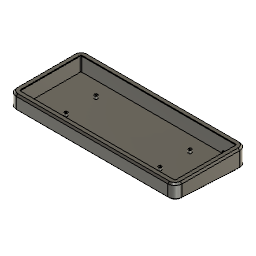
CNC QAZ MFR2 (Autodesk Fusion 360 design; units mm, degrees)
Autodesk Fusion 360 part; units mm, degrees
sketch "PCB Plane" plane through (0, 0, 0) normal (0, 0, 1) x (1, 0, 0)
  line L0 (0, 0) -> (195.263, 0) construction
  line L1 (195.263, 0) -> (195.263, 76.2) construction
  line L2 (195.263, 76.2) -> (0, 76.2) construction
  line L3 (0, 76.2) -> (0, 0) construction
  line L4 (-0.5, -0.5) -> (195.763, -0.5)
  line L5 (195.763, -0.5) -> (195.763, 76.7)
  line L6 (195.763, 76.7) -> (-0.5, 76.7)
  line L7 (-0.5, 76.7) -> (-0.5, -0.5)
  line L8 (-7.5, 83.7) -> (-7.5, -7.5)
  line L9 (-7.5, -7.5) -> (202.763, -7.5)
  line L10 (202.763, -7.5) -> (202.763, 83.7)
  line L11 (202.763, 83.7) -> (-7.5, 83.7)
  dimension "d1" = 195.263
  dimension "d2" = 76.2
  dimension "d3" = 0.5
  dimension "d4" = 7.5
  constraint horizontal L0
  constraint vertical L1
  constraint horizontal L2
  constraint vertical L3
  constraint coincident L0.start L3.end
  measures "d1" distance of L0.start L0.end
  measures "d2" distance of L0.start L2.end
ref_plane "WorkPlane1" through (97.6315, 38.1, -3.46) normal (0, 0, 1) x (1, 0, 0)
ref_plane "WorkPlane2" through (97.6315, 38.1, 14.6) normal (0, 0, 1) x (1, 0, 0)
extrude "Extrude1" add sketch "PCB Plane" along normal up to surface (14.6 mm away) and the other way up to surface (3.46 mm away)
sketch "Angle Sketch" plane through (202.763, 0, 0) normal (1, 0, 0) x (0, 1, 0)
  line L0 (83.7, 14.6) -> (-7.5, 14.6)
  line L1 (-7.5, 14.6) -> (-7.5, -3.46)
  line L2 (-7.5, -3.46) -> (83.7, -3.46)
  line L3 (83.7, -3.46) -> (83.7, 14.6)
  line L4 (-7.5, 14.6) -> (-7.5, -3.6755)
  line L5 (-7.5, -3.6755) -> (92.363, -8.9091)
  line L6 (-7.5, -3.6755) -> (92.5, -3.6755) construction
  dimension "d11" = 18.2755
  dimension "d12" = 100
  dimension "d13" = 3
  constraint coincident L0.end L1.start
  constraint perpendicular L0 L4
  constraint horizontal L6
  measures "d11" distance of L0.end L4.end
  measures "d12" distance of L4.end L5.end
  measures "d13" angle of L5 L6
ref_plane "WorkPlane3" through (202.763, 42.4315, -6.2923) normal (0, -0.052336, -0.99863) x (0, 0.99863, -0.052336)
sketch "Interior Base Plane" plane through (0, 0, -3.46) normal (0, 0, -1) x (1, 0, 0)
  line L0 (195.763, -76.7) -> (-0.5, -76.7)
  line L1 (-0.5, -76.7) -> (-0.5, 0.5)
  line L2 (-0.5, 0.5) -> (195.763, 0.5)
  line L3 (195.763, 0.5) -> (195.763, -76.7)
  line L4 (-7.5, 7.5) -> (-7.5, -83.7)
  line L5 (-7.5, -83.7) -> (202.763, -83.7)
  line L6 (202.763, -83.7) -> (202.763, 7.5)
  line L7 (202.763, 7.5) -> (-7.5, 7.5)
  line L8 (-7.5, 7.5) -> (202.763, 7.5)
  line L9 (202.763, 7.5) -> (202.763, -83.7)
  line L10 (202.763, -83.7) -> (-7.5, -83.7)
  line L11 (-7.5, -83.7) -> (-7.5, 7.5)
  constraint horizontal L8
  constraint vertical L9
  constraint horizontal L10
  constraint vertical L11
  constraint coincident L5.end L6.start
  constraint coincident L4.start L7.end
extrude "Extrude2" add sketch "Interior Base Plane" along normal up to surface contours L0 L1 L2 L3 | L4 L5 L6 L7 L8 L9 L10 L11 end surface through (202.763, 42.4315, -6.2923) normal (0, -0.052336, -0.99863) offset 0
fillet "Fillet1" radius 9 1 edges at (202.763, -7.5, 5.4623)
fillet "Fillet2" radius 9 1 edges at (202.763, 83.7, 3.0725)
fillet "Fillet3" radius 9 1 edges at (-7.5, 83.7, 3.0725)
fillet "Fillet4" radius 9 1 edges at (-7.5, -7.5, 5.4623)
fillet "Fillet5" radius 1 1 edges at (195.763, 76.7, 5.57)
fillet "Fillet6" radius 1 1 edges at (-0.5, 76.7, 5.57)
fillet "Fillet7" radius 1 1 edges at (195.763, -0.5, 5.57)
fillet "Fillet8" radius 1 1 edges at (-0.5, -0.5, 5.57)
chamfer "Chamfer1" distance 2 angle 45 8 edges at (-7.5, 38.1, 14.6) (-4.864, 81.064, 14.6) (97.6315, 83.7, 14.6) (200.127, 81.064, 14.6) (202.763, 38.1, 14.6) (200.127, -4.864, 14.6) (97.6315, -7.5, 14.6) (-4.864, -4.864, 14.6)
chamfer "Chamfer2" distance 2 angle 45 8 edges at (-7.5, 38.1, -6.0653) (-4.864, -4.864, -3.8136) (97.6315, -7.5, -3.6755) (200.127, -4.864, -3.8136) (202.763, 38.1, -6.0653) (200.127, 81.064, -8.3169) (97.6315, 83.7, -8.4551) (-4.864, 81.064, -8.3169)
chamfer "Chamfer3" distance 0.5 angle 45 4 edges at (97.6315, 76.7, 14.6) (-0.5, 38.1, 14.6) (97.6315, -0.5, 14.6) (195.763, 38.1, 14.6)
extrude "Extrude3" add 1 faces at (129.6753, 23.5658, -5.3036) along direction (0, 0.052336, 0.99863) blind 1
ref_plane "WorkPlane4" through (97.6315, 38.1, 0) normal (0, 0, 1) x (1, 0, 0)
sketch "USB C Hole Internal" plane through (0, 76.7, 0) normal (0, -1, 0) x (1, 0, 0)
  line L0 (194.763, 14.1) -> (0.5, 14.1)
  line L1 (0.5, -3.46) -> (194.763, -3.46)
  line L2 (180.1818, -3.46) -> (186.5317, -3.46)
  line L3 (188.0818, -1.91) -> (188.0818, -1.35)
  line L4 (186.5318, 0.2) -> (180.1818, 0.2)
  line L5 (178.6318, -1.35) -> (178.6318, -1.91)
  arc A0 (180.1818, 0.2) -> (178.6318, -1.35) centre (180.1818, -1.35) ccw
  arc A1 (188.0818, -1.35) -> (186.5318, 0.2) centre (186.5318, -1.35) ccw
  arc A2 (186.5318, -3.46) -> (188.0818, -1.91) centre (186.5318, -1.91) ccw
  arc A3 (178.6318, -1.91) -> (180.1818, -3.46) centre (180.1818, -1.91) ccw
  line L6 (0.5, 14.1) -> (0.5, -3.46)
  line L7 (194.763, -3.46) -> (194.763, 14.1)
  line L8 (194.763, -0.2545) -> (195.263, -0.2545)
  line L9 (183.3568, 0.2) -> (183.3568, -3.46) construction
  dimension "d36" = 1.55
  dimension "d82" = 0.5
  dimension "d83" = 4.725
  dimension "d84" = 11.9062
  dimension "d89" = 3.66
  dimension "d90" = 3.66
  constraint horizontal L2
  constraint vertical L3
  constraint horizontal L4
  constraint vertical L5
  constraint tangent L5 A0
  constraint tangent L4 A0
  constraint tangent L4 A1
  constraint tangent L3 A1
  constraint equal A0 A1
  constraint tangent L2 A2
  constraint tangent L3 A2
  constraint equal A0 A2
  constraint tangent L2 A3
  constraint tangent L5 A3
  constraint equal A0 A3
  constraint coincident L7 L8.start
  constraint perpendicular L7 L8
  constraint midpoint L4 L9.start
  constraint midpoint L2 L9.end
  measures "d36" radius of A0
  measures "d82" distance of L8.start L8.end
  measures "d83" distance of L5 L9
  measures "d84" distance of L8.end L9
  measures "d89" distance of L2 L4
  measures "d90" distance of L1 L4
extrude "Extrude4" cut sketch "USB C Hole Internal" against normal through all contours L1 L2 L3 L4 L5 A0 A1 A2 A3
sketch "USB C Hole External" plane through (0, 83.7, 0) normal (0, 1, 0) x (-1, 0, 0)
  line L0 (-186.5318, 0.2) -> (-180.1818, 0.2)
  arc A0 (-178.6318, -1.35) -> (-180.1818, 0.2) centre (-180.1817, -1.35) ccw
  line L1 (-178.6318, -1.35) -> (-178.6318, -1.91)
  arc A1 (-180.1818, -3.46) -> (-178.6317, -1.91) centre (-180.1817, -1.91) ccw
  line L2 (-180.1818, -3.46) -> (-186.5317, -3.46)
  arc A2 (-188.0818, -1.91) -> (-186.5318, -3.46) centre (-186.5318, -1.91) ccw
  line L3 (-188.0818, -1.91) -> (-188.0818, -1.35)
  arc A3 (-186.5318, 0.2) -> (-188.0818, -1.35) centre (-186.5318, -1.35) ccw
  line L4 (-193.763, -6.4551) -> (-1.5, -6.4551)
  line L5 (-1.5, -6.4551) -> (-1.5, 12.6)
  line L6 (-1.5, 12.6) -> (-193.763, 12.6)
  line L7 (-193.763, 12.6) -> (-193.763, -6.4551)
  line L8 (-178.6318, -1.63) -> (-188.0817, -1.63) construction
  line L9 (-183.3568, 0.2) -> (-183.3568, -3.46) construction
  line L10 (-183.8568, 2.45) -> (-183.8568, -5.71) construction
  line L11 (-190.8318, -1.63) -> (-176.8818, -1.63) construction
  line L12 (-186.5318, 2.45) -> (-180.1818, 2.45)
  line L13 (-176.3818, -1.35) -> (-176.3818, -1.91)
  line L14 (-180.1818, -5.71) -> (-186.5318, -5.71)
  line L15 (-190.3318, -1.91) -> (-190.3318, -1.35)
  arc A4 (-190.3318, -1.91) -> (-186.5318, -5.71) centre (-186.5318, -1.91) ccw
  arc A5 (-186.5318, 2.45) -> (-190.3318, -1.35) centre (-186.5318, -1.35) ccw
  arc A6 (-176.3818, -1.35) -> (-180.1818, 2.45) centre (-180.1818, -1.35) ccw
  arc A7 (-180.1818, -5.71) -> (-176.3818, -1.91) centre (-180.1818, -1.91) ccw
  dimension "d39" = 8.16
  dimension "d40" = 4.08
  dimension "d42" = 13.95
  dimension "d43" = 3.8
  dimension "d85" = 13.95
  dimension "d86" = 8.16
  dimension "d87" = 6.975
  dimension "d88" = 4.08
  constraint midpoint L1 L8.start
  constraint midpoint L0 L9.start
  constraint midpoint L2 L9.end
  constraint perpendicular L2 L10
  constraint perpendicular L10 L11
  constraint horizontal L12
  constraint vertical L13
  constraint horizontal L14
  constraint vertical L15
  constraint tangent L14 A4
  constraint tangent L15 A4
  constraint tangent L15 A5
  constraint tangent L12 A5
  constraint equal A4 A5
  constraint tangent L12 A6
  constraint tangent L13 A6
  constraint equal A4 A6
  constraint tangent L13 A7
  constraint tangent L14 A7
  constraint equal A4 A7
  measures "d39" distance of L10.start L10.end
  measures "d40" distance of L8 L10.start
  measures "d42" distance of L11.start L11.end
  measures "d43" radius of A4
  measures "d85" distance of L13 L15
  measures "d86" distance of L12 L14
  measures "d87" distance of L9 L15
extrude "Extrude5" cut sketch "USB C Hole External" against normal blind 4.5025 contours L12 L13 L14 L15 A4 A5 A6 A7
chamfer "Chamfer4" distance 0.25 angle 45 8 edges at (189.2188, 83.7, -4.597) (190.3318, 83.7, -1.63) (189.2188, 83.7, 1.337) (183.3568, 83.7, 2.45) (177.4947, 83.7, 1.337) (176.3818, 83.7, -1.63) (177.4947, 83.7, -4.597) (183.3568, 83.7, -5.71)
sketch "Hole Tops" plane through (0, 0, 0) normal (0, 0, 1) x (1, 0, 0)
  line L0 (0, 0) -> (195.2625, 0) construction
  line L1 (195.2625, 0) -> (195.2625, 76.2) construction
  line L2 (195.2625, 76.2) -> (0, 76.2) construction
  line L3 (0, 76.2) -> (0, 0) construction
  line L4 (195.2625, 76.2) -> (195.2625, 57.15) construction
  line L5 (195.2625, 57.15) -> (193.1449, 57.15) construction
  circle A0 centre (157.1625, 57.15) radius 2
  circle A1 centre (38.1, 57.15) radius 2
  circle A2 centre (38.1, 19.05) radius 2
  circle A3 centre (157.1625, 19.05) radius 2
  dimension "d47" = 195.2625
  dimension "d48" = 76.2
  dimension "d51" = 19.05
  dimension "d52" = 38.1
  dimension "d53" = 19.05
  dimension "d54" = 38.1
  dimension "d55" = 38.1
  dimension "d56" = 19.05
  dimension "d57" = 38.1
  dimension "d58" = 19.05
  dimension "d59" = 4
  constraint horizontal L0
  constraint vertical L1
  constraint horizontal L2
  constraint vertical L3
  constraint coincident L0.start L3.end
  constraint perpendicular L2 L4
  constraint perpendicular L1 L5
  constraint equal A0 A1
  constraint equal A0 A3
  constraint equal A1 A2
  measures "d47" distance of L0.start L0.end
  measures "d48" distance of L0.start L2.end
  measures "d51" distance of L2 A0.centre
  measures "d52" distance of L1 A0.centre
  measures "d53" distance of L0 A3.centre
  measures "d54" distance of L1 A3.centre
  measures "d55" distance of L3 A2.centre
  measures "d56" distance of L0 A2.centre
  measures "d57" distance of L3 A1.centre
  measures "d58" distance of L2 A1.centre
  measures "d59" diameter of A1
extrude "Extrude6" add sketch "Hole Tops" against normal up to surface (3.46 mm away)
hole "Hole1" at (157.1625, 19.05, 0) direction (0, 0, -1) diameter 1.6 depth 4 tip angle 180
hole "Hole2" at (157.1625, 57.15, 0) direction (0, 0, -1) diameter 1.6 depth 4 tip angle 180
hole "Hole3" at (38.1, 19.05, 0) direction (0, 0, -1) diameter 1.6 depth 4 tip angle 180
hole "Hole4" at (38.1, 57.15, 0) direction (0, 0, -1) diameter 1.6 depth 4 tip angle 180
sketch "Sketch11" plane through (0, -0.2126, -4.0574) normal (0, -0.052336, -0.99863) x (1, 0, 0)
  line L0 (200.763, -74.9106) -> (200.763, -1.715)
  spline S0 degree 3 poles (200.7625, -1.6334) (200.7627, -1.647) (200.7628, -1.6606) (200.763, -1.6878) (200.763, -1.7014) (200.763, -1.715) knots 1.559167 1.559167 1.559167 1.559167 1.564981 1.564981 1.570796 1.570796 1.570796 1.570796
  spline S1 degree 3 poles (193.763, 5.2974) (194.9008, 5.2974) (196.0377, 5.0141) (197.6563, 4.154) (198.2207, 3.7362) (198.7118, 3.2445) (199.2028, 2.7527) (199.6203, 2.1873) (200.467, 0.5894) (200.7496, -0.52) (200.7625, -1.6334) knots 0 0 0 0 0.48784 0.48784 0.785398 0.785398 0.785398 1.082956 1.082956 1.559167 1.559167 1.559167 1.559167
  line L1 (193.763, 5.2974) -> (1.5, 5.2974)
  spline S2 degree 3 poles (-5.4995, -1.6334) (-5.4866, -0.52) (-5.204, 0.5894) (-4.3573, 2.1873) (-3.9398, 2.7527) (-3.4488, 3.2445) (-2.9577, 3.7362) (-2.3933, 4.154) (-0.7747, 5.0141) (0.3622, 5.2974) (1.5, 5.2974) knots -1.559167 -1.559167 -1.559167 -1.559167 -1.082956 -1.082956 -0.785398 -0.785398 -0.785398 -0.48784 -0.48784 0 0 0 0
  spline S3 degree 3 poles (-5.5, -1.715) (-5.5, -1.7014) (-5.5, -1.6878) (-5.4998, -1.6606) (-5.4997, -1.647) (-5.4995, -1.6334) knots -1.570796 -1.570796 -1.570796 -1.570796 -1.564981 -1.564981 -1.559167 -1.559167 -1.559167 -1.559167
  line L2 (-5.5, -1.715) -> (-5.5, -74.9106)
  line L3 (-5.5, -75.0154) -> (-5.5, -74.9106)
  spline S4 degree 3 poles (1.5, -82.0278) (0.3678, -82.0278) (-0.7633, -81.7474) (-2.384, -80.8913) (-2.9537, -80.4706) (-3.4488, -79.9749) (-3.9439, -79.4791) (-4.3641, -78.9085) (-5.2196, -77.2845) (-5.5, -76.1504) (-5.5, -75.0154) knots 0 0 0 0 0.485398 0.485398 0.785398 0.785398 0.785398 1.085398 1.085398 1.570796 1.570796 1.570796 1.570796
  line L4 (1.5, -82.0278) -> (193.763, -82.0278)
  spline S5 degree 3 poles (200.763, -75.0154) (200.763, -76.1504) (200.4826, -77.2845) (199.6271, -78.9085) (199.2069, -79.4791) (198.7118, -79.9749) (198.2167, -80.4706) (197.647, -80.8913) (196.0263, -81.7474) (194.8952, -82.0278) (193.763, -82.0278) knots -1.570796 -1.570796 -1.570796 -1.570796 -1.085398 -1.085398 -0.785398 -0.785398 -0.785398 -0.485398 -0.485398 0 0 0 0
  line L5 (200.763, -74.9106) -> (200.763, -75.0154)
  circle A0 centre (195.763, -77.0278) radius 3.25
  circle A1 centre (195.763, 0.2974) radius 3.25
  circle A2 centre (-0.5, -77.0278) radius 3.25
  circle A3 centre (-0.5, 0.2974) radius 3.25
  dimension "d106" = 6.5
  dimension "d107" = 5
  dimension "d108" = 5
  dimension "d109" = 5
  dimension "d110" = 5
  dimension "d111" = 5
  dimension "d112" = 5
  dimension "d113" = 5
  dimension "d114" = 5
  constraint equal A0 A1
  constraint equal A0 A2
  constraint equal A0 A3
  measures "d106" diameter of A0
  measures "d107" distance of L4 A0.centre
  measures "d108" distance of L0 A0.centre
  measures "d109" distance of L0 A1.centre
  measures "d110" distance of L1 A1.centre
  measures "d111" distance of L1 A3.centre
  measures "d112" distance of L2 A3.centre
  measures "d113" distance of L2 A2.centre
  measures "d114" distance of L4 A2.centre
extrude "Extrude8" cut sketch "Sketch11" against normal blind 0.5 contours A0 | A1 | A2 | A3
move_body "Move1" [suppressed]
equation "d87 = ( 13.95 / 2 ) * 1 mm"
equation "d88 = ( 8.16 / 2 ) * 1 mm"
equation "d108 = d107"
equation "d109 = d107"
equation "d110 = d107"
equation "d111 = d107"
equation "d112 = d107"
equation "d113 = d107"
equation "d114 = d107"
